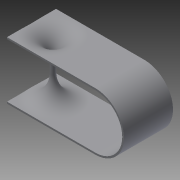
# Autodesk Inventor part: space time
Saved by Autodesk Inventor 2013 (Build 170138000, 138)
## iProperties
Created: 2012-11-30
Part Number: space time
Material: Generic
Document SubType Name: Modeling
Designer: Wilder
Density: 1 g/cm^3
Author: Wilder
Autodesk Inventor part; units mm, degrees
ref_plane "YZ Plane" through (0, 0, 0) normal (1, 0, 0) x (0, 1, 0)
ref_plane "XZ Plane" through (0, 0, 0) normal (0, 1, 0) x (-1, 0, 0)
ref_plane "XY Plane" through (0, 0, 0) normal (0, 0, 1) x (1, 0, 0)
sketch "Sketch1" plane through (0, 0, 0) normal (0, 0, 1) x (1, 0, 0)
  arc A0 (0, -5.6567) -> (0, 6.271) centre (-0.2268, 0.3072) ccw
  line L0 (0, 6.271) -> (-18.4804, 6.271)
  line L1 (0, -5.6567) -> (-18.4804, -5.6567)
  line L2 (-18.122, 5.9127) -> (-0.0069, 5.9127)
  arc A1 (-0.0069, -5.2984) -> (-0.0069, 5.9127) centre (-0.2268, 0.3072) ccw
  line L3 (-0.0069, -5.2984) -> (-18.122, -5.2984)
  line L4 (-18.122, 5.9127) -> (-18.4804, 5.9127)
  line L5 (-18.4804, 6.271) -> (-18.4804, 5.9127)
  line L6 (-18.122, -5.2984) -> (-18.4804, -5.2984)
  line L7 (-18.4804, -5.6567) -> (-18.4804, -5.2984)
  point P0 (0, 0)
  constraints: 16 end point, 4 point on circle, 3 parallel, 3 perpendicular, 2 centre point, 1 horizontal, 2 other
extrude "Extrusion1" add sketch "Sketch1" along normal blind 10.16
sketch "Sketch2" plane through (-18.4804, -5.2984, 0) normal (0, 1, 0) x (1, 0, 0)
  circle A0 centre (4.4536, -5.08) radius 0.4915
  point P0 (18.4804, 0)
  constraints: 1 centre point
extrude "Extrusion2" add sketch "Sketch2" along normal blind 11.43
fillet "Fillet1" radius 4.7625 1 edges at (-14.5182, -5.2984, 5.08)
fillet "Fillet2" radius 4.7625 1 edges at (-14.5182, 5.9127, 5.08)
sketch "Sketch3" plane through (-18.4804, -5.6567, 0) normal (0, -1, 0) x (1, 0, 0)
  circle A0 centre (4.4536, 5.08) radius 0.399
  constraints: 1 centre point
extrude "Extrusion3" cut sketch "Sketch3" against normal blind 25.4
fillet "Fillet3" radius 4.7625 1 edges at (-14.4258, 6.271, 5.08)
fillet "Fillet4" radius 4.7625 1 edges at (-14.4258, -5.6567, 5.08)
body "Solid1"
